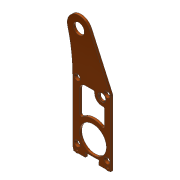
# Autodesk Inventor part: UPPER_LEG_MIDDLE_FRAME
Saved by Autodesk Inventor 2019.4 (Build 234330000, 330)
## iProperties
Created: 2019-11-13
Part Number: UPPER_LEG_MIDDLE_FRAME
Material: 一般
Document SubType Name: Modeling
Designer: y6tada
Density: 1 g/cm^3
Appearance: 滑らか - 淡いオレンジ
Author: y6tada
Autodesk Inventor part; units mm, degrees
ref_plane "YZ Plane" through (0, 0, 0) normal (1, 0, 0) x (0, 1, 0)
ref_plane "XZ Plane" through (0, 0, 0) normal (0, 1, 0) x (-1, 0, 0)
ref_plane "XY Plane" through (0, 0, 0) normal (0, 0, 1) x (1, 0, 0)
sketch "スケッチ1" plane through (0, 0, 0) normal (0, 0, 1) x (1, 0, 0)
  circle A0 centre (13.5, 29.015) radius 1.3 construction
  circle A1 centre (-13.5, 29.015) radius 1.3 construction
  circle A2 centre (-13.5, -22.985) radius 1.3 construction
  circle A3 centre (13.5, -22.985) radius 1.3 construction
  line L0 (13.5, 29.015) -> (-13.5, 29.015) construction
  line L1 (-13.5, 29.015) -> (-13.5, -22.985) construction
  line L2 (-13.5, -22.985) -> (13.5, -22.985) construction
  line L3 (13.5, -22.985) -> (13.5, 29.015) construction
  line L4 (21.1178, -22.6697) -> (19.2418, 24.6807)
  arc A4 (19.2418, 24.6807) -> (18.3199, 28.5854) centre (8.75, 24.265) ccw
  line L5 (0, 0) -> (0, -35.9566) construction
  circle A5 centre (-12.061, 67.9318) radius 5
  line L6 (-16.75, -30.235) -> (-15.5, -30.235) projected
  arc A6 (-15.5, -30.235) -> (-12.5, -30.235) centre (-14, -28.235) ccw projected
  line L7 (-12.5, -30.235) -> (-6.1, -30.235) projected
  line L8 (-6.1, -30.235) -> (-6.1, -27.6492) projected
  arc A7 (-4.6858, -26.235) -> (-6.1, -27.6492) centre (-5.3929, -26.9421) ccw projected
  line L9 (-4.6858, -26.235) -> (4.6858, -26.235) projected
  arc A8 (6.1, -27.6492) -> (4.6858, -26.235) centre (5.3929, -26.9421) ccw projected
  line L10 (6.1, -27.6492) -> (6.1, -30.235) projected
  line L11 (6.1, -30.235) -> (12.5, -30.235) projected
  arc A9 (12.5, -30.235) -> (15.5, -30.235) centre (14, -28.235) ccw projected
  line L12 (15.5, -30.235) -> (16.75, -30.235) projected
  arc A10 (-11.25, -10.8278) -> (11.25, -6.4392) centre (0.8, -12.735) ccw construction
  circle A11 centre (0.8, -12.735) radius 12.2
  circle A12 centre (-12.061, 67.9318) radius 5 construction
  circle A13 centre (8.75, 24.265) radius 3 construction
  line L13 (-11.25, 1.4772) -> (-11.25, 21.265)
  arc A14 (-6.25, 26.265) -> (-11.25, 21.265) centre (-6.25, 21.265) ccw
  line L14 (-6.25, 26.265) -> (1.25, 26.265)
  line L15 (11.25, 16.765) -> (11.25, 2.5355)
  arc A15 (2.25, 24.265) -> (8.75, 17.765) centre (8.75, 24.265) ccw
  line L16 (8.75, 17.765) -> (10.25, 17.765)
  line L17 (2.25, 24.265) -> (2.25, 25.265)
  arc A16 (11.25, 16.765) -> (10.25, 17.765) centre (10.25, 16.765) ccw
  arc A17 (2.25, 25.265) -> (1.25, 26.265) centre (1.25, 25.265) ccw
  arc A18 (8.9915, 1.2414) -> (-8.8559, 0.2728) centre (0.8, -12.735) ccw
  arc A19 (8.9915, 1.2414) -> (11.25, 2.5355) centre (9.75, 2.5355) ccw
  arc A20 (-11.25, 1.4772) -> (-8.8559, 0.2728) centre (-9.75, 1.4772) ccw
  line L18 (18.3199, 28.5854) -> (-1.5796, 72.6637)
  arc A21 (-1.5796, 72.6637) -> (-23.0621, 64.5812) centre (-12.061, 67.9318) ccw
  line L19 (-18.25, -25.6185) -> (-16.75, -30.235)
  line L20 (16.75, -30.235) -> (21.1178, -22.6697)
  line L21 (16.0414, 27.5568) -> (-3.8582, 71.635) construction
  arc A22 (16.7437, 24.5817) -> (16.0414, 27.5568) centre (8.75, 24.265) ccw construction
  line L22 (18.7764, -26.7219) -> (16.7437, 24.5817) construction
  arc A23 (-15.75, 32.265) -> (-20.6705, 65.3096) centre (-129.1686, 32.265) ccw construction
  line L23 (-15.75, 32.265) -> (-15.75, -31.3287) construction
  line L24 (-18.25, -25.6185) -> (-18.25, 32.265)
  arc A24 (-18.25, 32.265) -> (-23.0621, 64.5812) centre (-129.1686, 32.265) ccw
  point P0 (0, -56.485)
  point P1 (11.25, -0.3561)
  point P2 (-11.25, -1.9074)
  dimension "d3" = 10
  dimension "d22" = 3.5
  dimension "d23" = 1
  dimension "d24" = 1.5
  dimension "d25" = 4
  dimension "d35" = 11.5
  dimension "d37" = 18
  dimension "d38" = 30
  constraints: 36 end point, 26 point on circle, 16 centre point, 15 tangent, 9 coincident, 5 parallel, 4 vertical, 3 equal radius, 2 concentric, 2 horizontal, 2 perpendicular, 2 point on line, 25 other
  measures "d3" diameter of A5
  measures "d22" radial gap between concentric circles of A15 A13
  measures "d23" radius of A16
  measures "d24" radius of A19
  measures "d25" radial gap between concentric circles of A11 A18
  measures "d35" radius of A21
  measures "d37" angle of L19 L23
  measures "d38" angle of L3 L20
extrude "押し出し1" add sketch "スケッチ1" against normal blind 2
hole "穴1" at (-13.5, 29.015, 0) at (-13.5, -22.985, 0) at (13.5, -22.985, 0) at (13.5, 29.015, 0) direction (0, 0, -1) diameter 2.9 end through all countersink diameter 5.5 countersink angle 90 clearance for "Countersunk Flat Head Screw ISO 2009/7046" size "M2.5" standard "ISO"
hole "穴2" at (14, -28.235, 0) at (-14, -28.235, 0) direction (0, 0, -1) diameter 2 end through all
hole "穴3" at (8.75, 24.265, 0) direction (0, 0, -1) diameter 6 end through all counterbore diameter 7.3 counterbore depth 0.65
